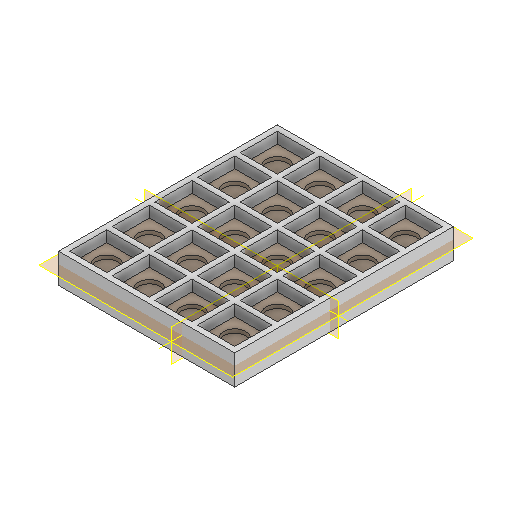
# Autodesk Inventor part: PanHolder
Saved by Autodesk Inventor 2025.1 (Build 291241000, 241)
## iProperties
Created: 2025-06-04
Part Number: PanHolder
Material: Generic
Document SubType Name: Modeling
Designer: Emlyn
Density: 1 g/cm^3
Appearance: Default
Author: Emlyn
Autodesk Inventor part; units mm, degrees
sketch "Sketch1" plane through (0, 0, 0) normal (0, 1, 0) x (-1, 0, 0)
  line L0 (-14.2136, -33.3126) -> (33.2864, -33.3126)
  line L1 (33.2864, -33.3126) -> (33.2864, 25.6874)
  line L2 (33.2864, 25.6874) -> (-14.2136, 25.6874)
  line L3 (-14.2136, 25.6874) -> (-14.2136, -33.3126)
  point P0 (0, 0)
  dimension "d0" = 59
  dimension "d1" = 47.5
  constraints: 8 end point, 2 parallel, 1 horizontal, 1 perpendicular
  measures "d0" distance of L2.end L0.start
  measures "d1" distance of L1.end L2.end
extrude "Extrusion1" add sketch "Sketch1" against normal blind 5
sketch "Sketch2" plane through (0, 0, 0) normal (0, 1, 0) x (1, 0, 0)
  line L0 (-33.2864, 33.3126) -> (14.2136, 33.3126) projected
  line L1 (14.2136, 33.3126) -> (-33.2864, 33.3126)
  line L2 (-33.2864, 33.3126) -> (-33.2864, 31.8126)
  line L3 (-33.2864, 31.8126) -> (14.2136, 31.8126)
  line L4 (14.2136, 31.8126) -> (14.2136, 33.3126)
  line L5 (14.2136, 31.8126) -> (12.7136, 31.8126)
  line L6 (12.7136, 31.8126) -> (12.7136, 21.8126)
  line L7 (12.7136, 21.8126) -> (14.2136, 21.8126)
  line L8 (14.2136, 21.8126) -> (14.2136, 31.8126)
  line L9 (2.7136, 21.8126) -> (2.7136, 31.8126)
  line L10 (1.2136, 31.8126) -> (1.2136, 21.8126)
  line L11 (1.2136, 21.8126) -> (2.7136, 21.8126)
  line L12 (-8.7864, 21.8126) -> (-8.7864, 31.8126)
  line L13 (-10.2864, 31.8126) -> (-10.2864, 21.8126)
  line L14 (-10.2864, 21.8126) -> (-8.7864, 21.8126)
  line L15 (-20.2864, 21.8126) -> (-20.2864, 31.8126)
  line L16 (-21.7864, 31.8126) -> (-21.7864, 21.8126)
  line L17 (-21.7864, 21.8126) -> (-20.2864, 21.8126)
  line L18 (-31.7864, 21.8126) -> (-31.7864, 31.8126)
  line L19 (-33.2864, 31.8126) -> (-33.2864, 21.8126)
  line L20 (-33.2864, 21.8126) -> (-31.7864, 21.8126)
  line L21 (14.2136, 10.3126) -> (14.2136, 20.3126)
  line L22 (12.7136, 20.3126) -> (12.7136, 10.3126)
  line L23 (14.2136, 21.8126) -> (-33.2864, 21.8126)
  line L24 (-33.2864, 20.3126) -> (14.2136, 20.3126)
  line L25 (14.2136, 20.3126) -> (14.2136, 21.8126)
  line L26 (-33.2864, 21.8126) -> (-33.2864, 20.3126)
  line L27 (-33.2864, 20.3126) -> (-33.2864, 10.3126)
  line L28 (-31.7864, 10.3126) -> (-31.7864, 20.3126)
  line L29 (-21.7864, 20.3126) -> (-21.7864, 10.3126)
  line L30 (-20.2864, 10.3126) -> (-20.2864, 20.3126)
  line L31 (-10.2864, 20.3126) -> (-10.2864, 10.3126)
  line L32 (-8.7864, 10.3126) -> (-8.7864, 20.3126)
  line L33 (1.2136, 20.3126) -> (1.2136, 10.3126)
  line L34 (2.7136, 10.3126) -> (2.7136, 20.3126)
  line L35 (1.2136, 10.3126) -> (2.7136, 10.3126)
  line L36 (-10.2864, 10.3126) -> (-8.7864, 10.3126)
  line L37 (12.7136, 10.3126) -> (14.2136, 10.3126)
  line L38 (-33.2864, 10.3126) -> (-31.7864, 10.3126)
  line L39 (-21.7864, 10.3126) -> (-20.2864, 10.3126)
  line L40 (14.2136, -1.1874) -> (14.2136, 8.8126)
  line L41 (12.7136, 8.8126) -> (12.7136, -1.1874)
  line L42 (14.2136, 10.3126) -> (-33.2864, 10.3126)
  line L43 (-33.2864, 8.8126) -> (14.2136, 8.8126)
  line L44 (14.2136, 8.8126) -> (14.2136, 10.3126)
  line L45 (-33.2864, 10.3126) -> (-33.2864, 8.8126)
  line L46 (-33.2864, 8.8126) -> (-33.2864, -1.1874)
  line L47 (-31.7864, -1.1874) -> (-31.7864, 8.8126)
  line L48 (-21.7864, 8.8126) -> (-21.7864, -1.1874)
  line L49 (-20.2864, -1.1874) -> (-20.2864, 8.8126)
  line L50 (-10.2864, 8.8126) -> (-10.2864, -1.1874)
  line L51 (-8.7864, -1.1874) -> (-8.7864, 8.8126)
  line L52 (1.2136, 8.8126) -> (1.2136, -1.1874)
  line L53 (2.7136, -1.1874) -> (2.7136, 8.8126)
  line L54 (1.2136, -1.1874) -> (2.7136, -1.1874)
  line L55 (-10.2864, -1.1874) -> (-8.7864, -1.1874)
  line L56 (12.7136, -1.1874) -> (14.2136, -1.1874)
  line L57 (-33.2864, -1.1874) -> (-31.7864, -1.1874)
  line L58 (-21.7864, -1.1874) -> (-20.2864, -1.1874)
  line L59 (14.2136, -12.6874) -> (14.2136, -2.6874)
  line L60 (12.7136, -2.6874) -> (12.7136, -12.6874)
  line L61 (14.2136, -1.1874) -> (-33.2864, -1.1874)
  line L62 (-33.2864, -2.6874) -> (14.2136, -2.6874)
  line L63 (14.2136, -2.6874) -> (14.2136, -1.1874)
  line L64 (-33.2864, -1.1874) -> (-33.2864, -2.6874)
  line L65 (-33.2864, -2.6874) -> (-33.2864, -12.6874)
  line L66 (-31.7864, -12.6874) -> (-31.7864, -2.6874)
  line L67 (-21.7864, -2.6874) -> (-21.7864, -12.6874)
  line L68 (-20.2864, -12.6874) -> (-20.2864, -2.6874)
  line L69 (-10.2864, -2.6874) -> (-10.2864, -12.6874)
  line L70 (-8.7864, -12.6874) -> (-8.7864, -2.6874)
  line L71 (1.2136, -2.6874) -> (1.2136, -12.6874)
  line L72 (2.7136, -12.6874) -> (2.7136, -2.6874)
  line L73 (1.2136, -12.6874) -> (2.7136, -12.6874)
  line L74 (-10.2864, -12.6874) -> (-8.7864, -12.6874)
  line L75 (12.7136, -12.6874) -> (14.2136, -12.6874)
  line L76 (-33.2864, -12.6874) -> (-31.7864, -12.6874)
  line L77 (-21.7864, -12.6874) -> (-20.2864, -12.6874)
  line L78 (14.2136, -24.1874) -> (14.2136, -14.1874)
  line L79 (12.7136, -14.1874) -> (12.7136, -24.1874)
  line L80 (14.2136, -12.6874) -> (-33.2864, -12.6874)
  line L81 (-33.2864, -14.1874) -> (14.2136, -14.1874)
  line L82 (14.2136, -14.1874) -> (14.2136, -12.6874)
  line L83 (-33.2864, -12.6874) -> (-33.2864, -14.1874)
  line L84 (-33.2864, -14.1874) -> (-33.2864, -24.1874)
  line L85 (-31.7864, -24.1874) -> (-31.7864, -14.1874)
  line L86 (-21.7864, -14.1874) -> (-21.7864, -24.1874)
  line L87 (-20.2864, -24.1874) -> (-20.2864, -14.1874)
  line L88 (-10.2864, -14.1874) -> (-10.2864, -24.1874)
  line L89 (-8.7864, -24.1874) -> (-8.7864, -14.1874)
  line L90 (1.2136, -14.1874) -> (1.2136, -24.1874)
  line L91 (2.7136, -24.1874) -> (2.7136, -14.1874)
  line L92 (1.2136, -24.1874) -> (2.7136, -24.1874)
  line L93 (-10.2864, -24.1874) -> (-8.7864, -24.1874)
  line L94 (12.7136, -24.1874) -> (14.2136, -24.1874)
  line L95 (-33.2864, -24.1874) -> (-31.7864, -24.1874)
  line L96 (-21.7864, -24.1874) -> (-20.2864, -24.1874)
  line L97 (-33.2864, -25.6874) -> (-33.2864, 33.3126) projected
  line L98 (14.2136, -24.1874) -> (-33.2864, -24.1874)
  line L99 (-33.2864, -24.1874) -> (-33.2864, -25.6874)
  line L100 (-33.2864, -25.6874) -> (14.2136, -25.6874)
  line L101 (14.2136, -25.6874) -> (14.2136, -24.1874)
  point P0 (0, 0)
  point P1 (13.4636, 31.8126)
  point P2 (13.4636, 21.8126)
  point P3 (1.9636, 21.8126)
  point P4 (-9.5364, 21.8126)
  point P5 (-21.0364, 21.8126)
  point P6 (-32.5364, 21.8126)
  point P7 (1.9636, 10.3126)
  point P8 (-9.5364, 10.3126)
  point P9 (13.4636, 10.3126)
  point P10 (-32.5364, 10.3126)
  point P11 (-21.0364, 10.3126)
  point P12 (1.9636, -1.1874)
  point P13 (-9.5364, -1.1874)
  point P14 (13.4636, -1.1874)
  point P15 (-32.5364, -1.1874)
  point P16 (-21.0364, -1.1874)
  point P17 (1.9636, -12.6874)
  point P18 (-9.5364, -12.6874)
  point P19 (13.4636, -12.6874)
  point P20 (-32.5364, -12.6874)
  point P21 (-21.0364, -12.6874)
  point P22 (1.9636, -24.1874)
  point P23 (-9.5364, -24.1874)
  point P24 (13.4636, -24.1874)
  point P25 (-32.5364, -24.1874)
  point P26 (-21.0364, -24.1874)
  point P27 (12.7136, 21.8126)
  point P28 (2.7136, 21.8126)
  point P29 (1.2136, 21.8126)
  point P30 (-8.7864, 31.8126)
  point P31 (-10.2864, 21.8126)
  point P32 (-20.2864, 21.8126)
  point P33 (-20.2864, 31.8126)
  point P34 (-21.7864, 31.8126)
  point P35 (-21.7864, 21.8126)
  point P36 (-31.7864, 21.8126)
  point P37 (-31.7864, 31.8126)
  point P38 (-21.7864, -14.1874)
  point P39 (-21.7864, -24.1874)
  point P40 (-31.7864, -24.1874)
  point P41 (-10.2864, -24.1874)
  point P42 (-20.2864, -24.1874)
  point P43 (-20.2864, -14.1874)
  point P44 (1.2136, -14.1874)
  point P45 (-8.7864, -24.1874)
  point P46 (2.7136, -14.1874)
  point P47 (12.7136, -14.1874)
  point P48 (2.7136, -24.1874)
  point P49 (-21.7864, -2.6874)
  point P50 (-21.7864, -12.6874)
  point P51 (-31.7864, -12.6874)
  point P52 (-10.2864, -2.6874)
  point P53 (-10.2864, -12.6874)
  point P54 (-20.2864, -12.6874)
  point P55 (-20.2864, -2.6874)
  point P56 (1.2136, -2.6874)
  point P57 (1.2136, -12.6874)
  point P58 (-8.7864, -12.6874)
  point P59 (2.7136, -2.6874)
  point P60 (12.7136, -2.6874)
  point P61 (12.7136, -12.6874)
  point P62 (2.7136, -12.6874)
  point P63 (-21.7864, 8.8126)
  point P64 (-21.7864, -1.1874)
  point P65 (-31.7864, -1.1874)
  point P66 (-10.2864, -1.1874)
  point P67 (-20.2864, -1.1874)
  point P68 (-20.2864, 8.8126)
  point P69 (1.2136, 8.8126)
  point P70 (1.2136, -1.1874)
  point P71 (-8.7864, -1.1874)
  point P72 (2.7136, 8.8126)
  point P73 (12.7136, 8.8126)
  point P74 (12.7136, -1.1874)
  point P75 (2.7136, -1.1874)
  point P76 (-21.7864, 20.3126)
  point P77 (-21.7864, 10.3126)
  point P78 (-31.7864, 10.3126)
  point P79 (-20.2864, 10.3126)
  point P80 (-20.2864, 20.3126)
  point P81 (1.2136, 20.3126)
  point P82 (1.2136, 10.3126)
  point P83 (2.7136, 20.3126)
  point P84 (12.7136, 20.3126)
  point P85 (12.7136, 10.3126)
  point P86 (2.7136, 10.3126)
  point P87 (-33.2864, -24.1874)
  point P88 (-33.2864, -1.1874)
  point P89 (-33.2864, 10.3126)
  point P90 (-33.2864, 21.8126)
  point P91 (-33.2864, 31.8126)
  point P92 (-33.2864, -12.6874)
  dimension "d4" = 1.5
  dimension "d5" = 1.5
  dimension "d6" = 10
  dimension "d9" = 11.5
  dimension "d16" = 11.5
  constraints: 200 end point, 6 parallel, 4 horizontal, 3 perpendicular, 2 midpoint, 1 collinear, 1 vertical, 220 other
  measures "d4" distance between parallel lines of L3 L0
  measures "d5" distance between parallel lines of L6 L8
  measures "d6" distance of point (13.464, 31.813) point (13.464, 21.813)
  measures "d9" distance of L7.end L9.start
  measures "d16" distance of L7.end L21.start
extrude "Extrusion2" add sketch "Sketch2" along normal blind 3 contours L0 L4 L3 L2 | L3 L18 L20 L19 | L8 L7 L6 L3 | L20 L23 L17 L14 L11 L7 L25 L24 L26 | L3 L15 L17 L16 | L24 L28 L38 L27 | L9 L11 L10 L3 | L21 L37 L22 L24 | L38 L42 L39 L36 L35 L37 L44 L43 L45 | L3 L12 L14 L13 | L24 L30 L39 L29 | L43 L47 L57 L46 | L40 L56 L41 L43 | L34 L35 L33 L24 | L57 L61 L58 L55 L54 L56 L63 L62 L64 | L24 L32 L36 L31 | L43 L49 L58 L48 | L62 L66 L76 L65 | L59 L75 L60 L62 | L53 L54 L52 L43 | L76 L80 L77 L74 L73 L75 L82 L81 L83 | L43 L51 L55 L50 | L62 L68 L77 L67 | L81 L85 L95 L84 | L78 L94 L79 L81 | L72 L73 L71 L62 | L95 L98 L96 L93 L92 L94 L101 L100 L97 | L62 L70 L74 L69 | L81 L87 L96 L86 | L91 L92 L90 L81 | L81 L89 L93 L88
sketch "Sketch3" plane through (0, 0, 0) normal (0, 1, 0) x (1, 0, 0)
  circle A0 centre (-26.7864, 26.8126) radius 3
  line L0 (-21.7864, 31.8126) -> (-21.7864, 21.8126) projected
  line L1 (-31.7864, 31.8126) -> (-21.7864, 31.8126) projected
  circle A1 centre (-15.2864, 26.8126) radius 3
  circle A2 centre (-3.7864, 26.8126) radius 3
  circle A3 centre (7.7136, 26.8126) radius 3
  circle A4 centre (-26.7864, 15.3126) radius 3
  circle A5 centre (-15.2864, 15.3126) radius 3
  circle A6 centre (-3.7864, 15.3126) radius 3
  circle A7 centre (7.7136, 15.3126) radius 3
  circle A8 centre (-26.7864, 3.8126) radius 3
  circle A9 centre (-15.2864, 3.8126) radius 3
  circle A10 centre (-3.7864, 3.8126) radius 3
  circle A11 centre (7.7136, 3.8126) radius 3
  circle A12 centre (-26.7864, -7.6874) radius 3
  circle A13 centre (-15.2864, -7.6874) radius 3
  circle A14 centre (-3.7864, -7.6874) radius 3
  circle A15 centre (7.7136, -7.6874) radius 3
  circle A16 centre (-26.7864, -19.1874) radius 3
  circle A17 centre (-15.2864, -19.1874) radius 3
  circle A18 centre (-3.7864, -19.1874) radius 3
  circle A19 centre (7.7136, -19.1874) radius 3
  point P0 (0, 0)
  dimension "d23" = 6
  dimension "d24" = 5
  dimension "d25" = 5
  dimension "d28" = 11.5
  dimension "d31" = 11.5
  constraints: 20 centre point, 1 horizontal, 1 vertical, 38 other
  measures "d23" diameter of A0
  measures "d24" distance from line of L0 A0.centre
  measures "d25" distance from line of L1 A0.centre
  measures "d28" distance of A0.centre A1.centre
  measures "d31" distance of A0.centre A4.centre
extrude "Extrusion3" cut sketch "Sketch3" against normal blind 1
body "Solid1"
